Autodesk Fusion 360 part; units mm, degrees
(part 4 of 4)
sketch "Sketch10" plane through (-30.55, 0, 0) normal (-1, 0, 0) x (0, -1, 0)
  line L0 (-28.275, 0) -> (28.325, 0)
  line L1 (28.325, 0) -> (28.325, 20)
  line L2 (28.325, 20) -> (-28.275, 20)
  line L3 (-9.975, 15.25) -> (-9.975, 4.85)
  line L4 (14.525, 15.25) -> (14.525, 4.85)
  line L5 (-28.275, 20) -> (-28.275, 0)
  line L6 (-5.2906, 18) -> (9.8406, 18)
  line L7 (-5.2906, 2) -> (9.8406, 2)
  line L8 (-5.8274, 3.8437) -> (1.7382, 8.6576)
  line L9 (2.8118, 8.6576) -> (10.3774, 3.8437)
  line L10 (12.9967, 4.0009) -> (4.6396, 9.2009)
  line L11 (4.6396, 10.8991) -> (12.9967, 16.0991)
  line L12 (10.3774, 16.1563) -> (2.8118, 11.3424)
  line L13 (1.7382, 11.3424) -> (-5.8274, 16.1563)
  line L14 (-8.4467, 16.0991) -> (-0.0896, 10.8991)
  line L15 (-0.0896, 9.2009) -> (-8.4467, 4.0009)
  arc A0 (-8.4467, 16.0991) -> (-9.975, 15.25) centre (-8.975, 15.25) ccw
  arc A1 (-9.975, 4.85) -> (-8.4467, 4.0009) centre (-8.975, 4.85) ccw
  arc A2 (-0.0896, 9.2009) -> (-0.0896, 10.8991) centre (-0.6179, 10.05) ccw
  arc A3 (2.8118, 8.6576) -> (1.7382, 8.6576) centre (2.275, 7.8139) ccw
  arc A4 (9.8406, 2) -> (10.3774, 3.8437) centre (9.8406, 3) ccw
  arc A5 (-5.8274, 3.8437) -> (-5.2906, 2) centre (-5.2906, 3) ccw
  arc A6 (12.9967, 4.0009) -> (14.525, 4.85) centre (13.525, 4.85) ccw
  arc A7 (14.525, 15.25) -> (12.9967, 16.0991) centre (13.525, 15.25) ccw
  arc A8 (10.3774, 16.1563) -> (9.8406, 18) centre (9.8406, 17) ccw
  arc A9 (-5.2906, 18) -> (-5.8274, 16.1563) centre (-5.2906, 17) ccw
  arc A10 (1.7382, 11.3424) -> (2.8118, 11.3424) centre (2.275, 12.1861) ccw
  arc A11 (4.6396, 10.8991) -> (4.6396, 9.2009) centre (5.1679, 10.05) ccw
  line L16 (-28.275, 20) -> (-28.275, 0)
  point P0 (-9.975, 17.05)
  point P1 (-9.975, 3.05)
  point P2 (14.525, 17.05)
  point P3 (14.525, 3.05)
  point P4 (-8.725, 18)
  point P5 (13.275, 18)
  point P6 (-8.725, 2)
  point P7 (13.275, 2)
  point P8 (2.275, 10.05)
  dimension "d79" = 2
  dimension "d80" = 2
  dimension "d81" = 11
  dimension "d82" = 7
  dimension "d83" = 22
  dimension "d84" = 22
  dimension "d85" = 14
  dimension "d86" = 14
  dimension "d88" = 3.05
  dimension "d89" = 1
  dimension "d100" = 24.5
  dimension "d101" = 5.7857
  constraint perpendicular L2 L3
  constraint vertical L4
  constraint horizontal L6
  constraint perpendicular L3 L7
  constraint horizontal P0 P2
  constraint vertical P4 P6
  constraint coincident P0 L14
  constraint coincident P0 L3
  constraint tangent L14 A0
  constraint tangent L3 A0
  constraint coincident P1 L3
  constraint coincident P1 L15
  constraint tangent L3 A1
  constraint tangent L15 A1
  constraint equal A0 A1
  constraint tangent L15 A2
  constraint tangent L14 A2
  constraint equal A0 A2
  constraint tangent L8 A3
  constraint tangent L9 A3
  constraint equal A0 A3
  constraint coincident P7 L9
  constraint coincident P7 L7
  constraint tangent L9 A4
  constraint tangent L7 A4
  constraint equal A0 A4
  constraint coincident P6 L7
  constraint coincident P6 L8
  constraint tangent L7 A5
  constraint tangent L8 A5
  constraint equal A0 A5
  constraint coincident P3 L10
  constraint coincident P3 L4
  constraint tangent L10 A6
  constraint tangent L4 A6
  constraint equal A0 A6
  constraint coincident P2 L4
  constraint coincident P2 L11
  constraint tangent L4 A7
  constraint tangent L11 A7
  constraint equal A0 A7
  constraint coincident P5 L12
  constraint coincident P5 L6
  constraint tangent L12 A8
  constraint tangent L6 A8
  constraint equal A0 A8
  constraint coincident P4 L13
  constraint coincident P4 L6
  constraint tangent L13 A9
  constraint tangent L6 A9
  constraint equal A0 A9
  constraint tangent L13 A10
  constraint equal A0 A10
  constraint tangent L10 A11
  constraint tangent L11 A11
  constraint equal A0 A11
  constraint horizontal A0.centre A7.centre
  constraint horizontal A1.centre A6.centre
  constraint vertical A5.centre A9.centre
  constraint vertical A4.centre A8.centre
  constraint horizontal P8 A2.centre
  constraint vertical P8 A3.centre
  measures "d79" distance of L2 L6
  measures "d80" distance of L0 L7
  measures "d81" horizontal distance of P5 P8
  measures "d82" vertical distance of P2 P8
  measures "d83" distance of P4 P5
  measures "d84" distance of P6 P7
  measures "d85" distance of P2 P3
  measures "d86" distance of P0 P1
  measures "d88" distance of L0 P3
  measures "d89" radius of A0
  measures "d100" distance of L3 L4
  measures "d101" horizontal distance of A2.centre A11.centre
extrude "Extrude8" cut sketch "Sketch10" against normal blind 65 contours L3 L14 L15 A0 A1 A2 | L4 L10 L11 A6 A7 A11 | L6 L12 L13 A8 A9 A10 | L7 L8 L9 A3 A4 A5
extrude "Extrude9" cut 2 faces at (27.0333, 28.275, 6.6667) (-23.5167, 28.275, 13.3333) along direction (0, -1, 0) blind 1.55
extrude "Extrude10" cut 1 faces at (-17.3333, 38.275, 11.7192) along direction (0, -1, 0) blind 4.5
fillet "Fillet4" radius 2.5 6 edges at (-20, 26.725, 10) (-20, 33.775, 10) (-30.55, 26.725, 10) (20, 33.775, 10) (20, 26.725, 10) (30.55, 26.725, 10)
fillet "Fillet5" radius 2 2 edges at (-40.55, -29.575, 20) (40.55, -29.575, 20)
extrude "Extrude11" cut 2 faces at (-32.55, -30.825, 12.6667) (32.55, -30.825, 12.6667) along direction (0, 1, 0) blind 0.05
extrude "Extrude12" add 2 faces at (33.8833, -28.325, 12.6667) (-33.8833, -28.325, 12.6667) along direction (0, 1, 0) blind 7.55
sketch "Sketch11" plane through (0, -20.775, 0) normal (0, 1, 0) x (-1, 0, 0)
  arc A0 (-38.55, 20) -> (-40.55, 18) centre (-38.55, 18) ccw
  line L0 (-40.55, 18) -> (-40.55, 0)
  line L1 (-40.55, 0) -> (-30.55, 0)
  line L2 (-30.55, 0) -> (-30.55, 20)
  line L3 (-30.55, 20) -> (-38.55, 20)
  point P0 (-34.75, 10)
  point P1 (34.75, 10)
  dimension "d112" = 69.5
  dimension "d113" = 5.8
  dimension "d114" = 10
  constraint horizontal P0 P1
  measures "d112" distance of P0 P1
  measures "d113" distance of L0 P0
  measures "d114" distance of L3 P0
hole "Hole3" at (34.75, -20.775, 10) at (-34.75, -20.775, 10) direction (0, -1, 0) diameter 5.3 end through all counterbore diameter 10 counterbore depth 5
sketch "Sketch12" plane through (0, -20.775, 0) normal (0, 1, 0) x (-1, 0, 0)
  arc A0 (-30.55, 12.7129) -> (-30.55, 7.2871) centre (-34.75, 10) ccw
  line L0 (-30.55, 12.7129) -> (-30.55, 20)
  line L1 (-30.55, 20) -> (-38.55, 20)
  arc A1 (-38.55, 20) -> (-40.55, 18) centre (-38.55, 18) ccw
  line L2 (-40.55, 18) -> (-40.55, 0)
  line L3 (-40.55, 0) -> (-30.55, 0)
  line L4 (-30.55, 0) -> (-30.55, 7.2871)
  circle A2 centre (-34.75, 10) radius 5
  circle A3 centre (34.75, 10) radius 5
  dimension "d119" = 10
  dimension "d120" = 10
  dimension "d121" = 69.5
  constraint concentric A0 A2
  constraint horizontal A0.centre A3.centre
  measures "d119" diameter of A2
  measures "d120" diameter of A3
  measures "d121" distance of A0.centre A3.centre
extrude "Extrude13" cut sketch "Sketch12" along normal blind 7 contours A0 A2 | A3
equation "d4 = ( 52.55 / 2 ) * 1 mm"
equation "d8 = ( 57.1 / 2 ) * 1 mm"
equation "d88 = ( ( 20.1 - 14 ) / 2 ) * 1 mm"
equation "d99 = 57.55 mm + 1.55 mm"
equation "d110 = 10 mm - 2.45 mm"
